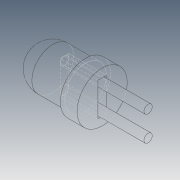
# Autodesk Inventor part: Led3mm
Saved by Autodesk Inventor 2015 (Build 190159000, 159)
## iProperties
Created: 2017-03-14
Part Number: Led3mm
Material: Generic
Document SubType Name: Modeling
Designer: Val
Density: 1 g/cm^3
Appearance: Default
Author: Val
Autodesk Inventor part; units mm, degrees
ref_plane "YZ Plane" through (0, 0, 0) normal (1, 0, 0) x (0, 1, 0)
ref_plane "XZ Plane" through (0, 0, 0) normal (0, 1, 0) x (-1, 0, 0)
ref_plane "XY Plane" through (0, 0, 0) normal (0, 0, 1) x (1, 0, 0)
sketch "Body" plane through (0, 0, 0) normal (0, 1, 0) x (-1, 0, 0)
  line L0 (0, 1.5) -> (0, 0)
  line L1 (0, 1.5) -> (1, 1.5)
  line L2 (1, 1.5) -> (1, 1.25)
  line L3 (0, 0) -> (4.2, 0)
  arc A0 (4.2, 0) -> (2.95, 1.25) centre (2.95, 0) ccw
  line L4 (2.95, 1.25) -> (1, 1.25)
  point P0 (0, 0)
  dimension "d1" = 1
  dimension "d2" = 4.2
  dimension "d3" = 1.5
  dimension "d4" = 0.25
  constraints: 10 end point, 2 horizontal, 2 perpendicular, 2 point on circle, 1 centre point, 1 coincident, 1 point on line, 1 tangent, 1 vertical
  measures "d1" distance of L0.start L1.end
  measures "d2" distance of L0.end L3.end
  measures "d3" distance of L0.start L0.end
  measures "d4" distance from line of L1.end L4
revolve "Revolution1" add sketch "Body" angle 360 about axis through (0, 0, 0) along (-1, 0, 0)
sketch "Sketch2" plane through (0, 0, 0) normal (1, 0, 0) x (0, 0, -1)
  line L0 (-1, 0.25) -> (1, 0.25)
  line L1 (1, 0.25) -> (1, -0.25)
  line L2 (1, -0.25) -> (-1, -0.25)
  line L3 (-1, -0.25) -> (-1, 0.25)
  circle A0 centre (0, 0) radius 1.5 construction
  line L4 (-1, 0) -> (1, 0) construction
  dimension "d9" = 0.5
  dimension "d10" = 0.5
  constraints: 10 end point, 3 midpoint, 2 parallel, 1 coincident, 1 horizontal, 1 perpendicular
  measures "d9" distance edge to line of A0 L3
  measures "d10" distance of L2.end L0.start
extrude "Extrusion1" cut sketch "Sketch2" against normal blind 2.25
sketch "Sketch3" plane through (-2.25, 0, 0) normal (1, 0, 0) x (0, 0, -1)
  circle A0 centre (-0.75, 0) radius 0.25
  line L0 (-1, 0.25) -> (1, 0.25) construction
  line L1 (1, -0.25) -> (-1, -0.25) construction
  line L2 (-1, -0.25) -> (-1, 0.25) projected
  line L3 (0, 0.25) -> (0, -0.25) construction
  circle A1 centre (0.75, 0) radius 0.25
  point P0 (0, 0)
  constraints: 3 tangent, 2 centre point, 2 end point, 2 midpoint, 1 symmetric about line, 1 other
extrude "Extrusion2" add sketch "Sketch3" along normal blind 5
body "Solid1"
